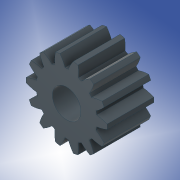
# Autodesk Inventor part: FA010
Saved by Autodesk Inventor 2017 SP1 (Build 210196100, 196)
## iProperties
Created: 2017-06-24
Part Number: FA010
Material: ABS Plastic
Document SubType Name: Modeling
Designer: Zach
Density: 1.06 g/cm^3
Appearance: CR Dark Blue
Author: Zach
Autodesk Inventor part; units mm, degrees
ref_plane "YZ Plane" through (0, 0, 0) normal (1, 0, 0) x (0, 1, 0)
ref_plane "XZ Plane" through (0, 0, 0) normal (0, 1, 0) x (-1, 0, 0)
ref_plane "XY Plane" through (0, 0, 0) normal (0, 0, 1) x (1, 0, 0)
sketch "Sketch1" plane through (0, 0, 0) normal (0, 0, 1) x (1, 0, 0)
  circle A0 centre (0, 0) radius 11.75
  circle A1 centre (0, 0) radius 5.5
  dimension "d0" = 23.5
  dimension "d1" = 11
  constraints: 2 centre point, 2 coincident
  measures "d0" diameter of A0
  measures "d1" diameter of A1
extrude "Extrusion1" add sketch "Sketch1" along normal blind 18
sketch "Sketch2" plane through (0, 0, 18) normal (0, 0, 1) x (1, 0, 0)
  line L0 (0, 0) -> (25, 0) construction
  circle A0 centre (0, 0) radius 11.75 construction
  arc A1 (15.5785, 0.9) -> (11.5785, 2) centre (9.6394, -12.8741) ccw
  arc A2 (15.5789, -0.9) -> (15.5785, 0.9) centre (-4.401, -0.0044) ccw
  arc A3 (11.5785, -2) -> (15.5789, -0.9) centre (9.64, 12.8742) ccw
  arc A4 (11.5785, -2) -> (11.5785, 2) centre (0, 0) ccw
  arc A5 (13.6453, 7.5701) -> (9.5641, 6.8257) centre (14.2707, -7.4168) ccw
  arc A6 (11.2997, 3.2218) -> (9.5641, 6.8257) centre (0, 0) ccw
  arc A7 (11.2997, 3.2218) -> (14.4266, 5.9486) centre (3.0994, 15.7819) ccw
  arc A8 (14.4266, 5.9486) -> (13.6453, 7.5701) centre (-3.9633, -1.9135) ccw
  arc A9 (9.0094, 12.7409) -> (5.6554, 10.2994) centre (16.0755, -0.4905) ccw
  arc A10 (8.7828, 7.8055) -> (5.6554, 10.2994) centre (0, 0) ccw
  arc A11 (8.7828, 7.8055) -> (10.417, 11.619) centre (-4.055, 15.5638) ccw
  arc A12 (10.417, 11.619) -> (9.0094, 12.7409) centre (-2.7405, -3.4436) ccw
  arc A13 (2.5891, 15.3882) -> (0.6266, 11.7333) centre (14.6963, 6.5329) ccw
  arc A14 (4.5263, 10.8432) -> (0.6266, 11.7333) centre (0, 0) ccw
  arc A15 (4.5263, 10.8432) -> (4.3441, 14.9881) centre (-10.4063, 12.2631) ccw
  arc A16 (4.3441, 14.9881) -> (2.5891, 15.3882) centre (-0.975, -4.2916) ccw
  arc A17 (-4.344, 14.9877) -> (-4.5263, 10.8432) centre (10.4064, 12.2625) ccw
  arc A18 (-0.6266, 11.7333) -> (-4.5263, 10.8432) centre (0, 0) ccw
  arc A19 (-0.6266, 11.7333) -> (-2.5892, 15.3886) centre (-14.6965, 6.5335) ccw
  arc A20 (-2.5892, 15.3886) -> (-4.344, 14.9877) centre (0.9836, -4.2897) ccw
  arc A21 (-10.4167, 11.6187) -> (-8.7828, 7.8055) centre (4.0553, 15.5633) ccw
  arc A22 (-5.6554, 10.2994) -> (-8.7828, 7.8055) centre (0, 0) ccw
  arc A23 (-5.6554, 10.2994) -> (-9.0097, 12.7412) centre (-16.0759, -0.4901) ccw
  arc A24 (-9.0097, 12.7412) -> (-10.4167, 11.6187) centre (2.7474, -3.4381) ccw
  arc A25 (-14.4263, 5.9484) -> (-11.2997, 3.2218) centre (-3.0989, 15.7816) ccw
  arc A26 (-9.5641, 6.8257) -> (-11.2997, 3.2218) centre (0, 0) ccw
  arc A27 (-9.5641, 6.8257) -> (-13.6456, 7.5703) centre (-14.2712, -7.4166) ccw
  arc A28 (-13.6456, 7.5703) -> (-14.4263, 5.9484) centre (3.9671, -1.9056) ccw
  arc A29 (-15.5785, -0.9) -> (-11.5785, -2) centre (-9.6394, 12.8741) ccw
  arc A30 (-11.5785, 2) -> (-11.5785, -2) centre (0, 0) ccw
  arc A31 (-11.5785, 2) -> (-15.5789, 0.9) centre (-9.64, -12.8742) ccw
  arc A32 (-15.5789, 0.9) -> (-15.5785, -0.9) centre (4.401, 0.0044) ccw
  arc A33 (-13.6453, -7.5701) -> (-9.5641, -6.8257) centre (-14.2707, 7.4168) ccw
  arc A34 (-11.2997, -3.2218) -> (-9.5641, -6.8257) centre (0, 0) ccw
  arc A35 (-11.2997, -3.2218) -> (-14.4266, -5.9486) centre (-3.0994, -15.7819) ccw
  arc A36 (-14.4266, -5.9486) -> (-13.6453, -7.5701) centre (3.9633, 1.9135) ccw
  arc A37 (-9.0094, -12.7409) -> (-5.6554, -10.2994) centre (-16.0755, 0.4905) ccw
  arc A38 (-8.7828, -7.8055) -> (-5.6554, -10.2994) centre (0, 0) ccw
  arc A39 (-8.7828, -7.8055) -> (-10.417, -11.619) centre (4.055, -15.5638) ccw
  arc A40 (-10.417, -11.619) -> (-9.0094, -12.7409) centre (2.7405, 3.4436) ccw
  arc A41 (-2.5891, -15.3882) -> (-0.6266, -11.7333) centre (-14.6963, -6.5329) ccw
  arc A42 (-4.5263, -10.8432) -> (-0.6266, -11.7333) centre (0, 0) ccw
  arc A43 (-4.5263, -10.8432) -> (-4.3441, -14.9881) centre (10.4063, -12.2631) ccw
  arc A44 (-4.3441, -14.9881) -> (-2.5891, -15.3882) centre (0.975, 4.2916) ccw
  arc A45 (4.344, -14.9877) -> (4.5263, -10.8432) centre (-10.4064, -12.2625) ccw
  arc A46 (0.6266, -11.7333) -> (4.5263, -10.8432) centre (0, 0) ccw
  arc A47 (0.6266, -11.7333) -> (2.5892, -15.3886) centre (14.6965, -6.5335) ccw
  arc A48 (2.5892, -15.3886) -> (4.344, -14.9877) centre (-0.9836, 4.2897) ccw
  arc A49 (10.4167, -11.6187) -> (8.7828, -7.8055) centre (-4.0553, -15.5633) ccw
  arc A50 (5.6554, -10.2994) -> (8.7828, -7.8055) centre (0, 0) ccw
  arc A51 (5.6554, -10.2994) -> (9.0097, -12.7412) centre (16.0759, 0.4901) ccw
  arc A52 (9.0097, -12.7412) -> (10.4167, -11.6187) centre (-2.7474, 3.4381) ccw
  arc A53 (14.4263, -5.9484) -> (11.2997, -3.2218) centre (3.0989, -15.7816) ccw
  arc A54 (9.5641, -6.8257) -> (11.2997, -3.2218) centre (0, 0) ccw
  arc A55 (9.5641, -6.8257) -> (13.6456, -7.5703) centre (14.2712, 7.4166) ccw
  arc A56 (13.6456, -7.5703) -> (14.4263, -5.9484) centre (-3.9671, 1.9056) ccw
  point P0 (15.599, 0)
  point P1 (14.0542, 6.7682)
  point P2 (9.7258, 12.1958)
  point P3 (3.4711, 15.2079)
  point P4 (-3.4711, 15.2079)
  point P5 (-9.7258, 12.1958)
  point P6 (-14.0542, 6.7682)
  point P7 (-15.599, 0)
  point P8 (-14.0542, -6.7682)
  point P9 (-9.7258, -12.1958)
  point P10 (-3.4711, -15.2079)
  point P11 (3.4711, -15.2079)
  point P12 (9.7258, -12.1958)
  point P13 (14.0542, -6.7682)
  dimension "d4" = 25
  dimension "d5" = 15
  dimension "d6" = 4
  dimension "d7" = 2
  dimension "d8" = 20
  dimension "d9" = 1.8
  dimension "d10" = 15
  dimension "d11" = 2
  dimension "d12" = 4.0004
  dimension "d15" = 360
  constraints: 115 point on circle, 56 centre point, 2 end point, 1 concentric, 1 horizontal, 1 point on line, 183 other
  measures "d4" distance of L0.start L0.end
  measures "d5" radius of A1
  measures "d6" horizontal distance of A1.start A0.start
  measures "d7" distance from line of L0 A0.start
  measures "d8" radius of A2
  measures "d9" distance of A2.start A1.start
  measures "d10" radius of A3
  measures "d11" distance from line of L0 A0.end
  measures "d12" horizontal distance of A0.end A2.start
extrude "Extrusion2" add sketch "Sketch2" against normal blind 18
body "Solid1"
